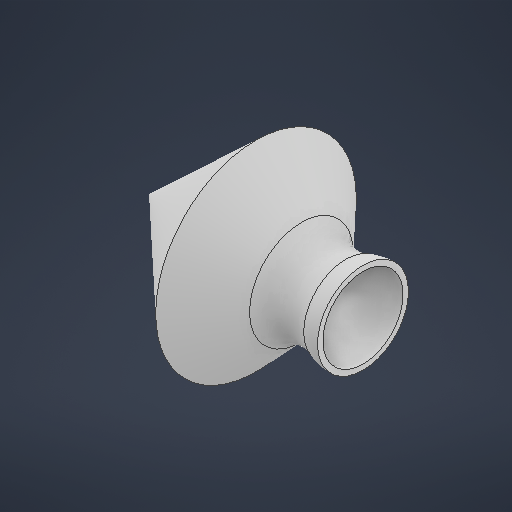
# Autodesk Inventor part: cabeza
Saved by Autodesk Inventor 2026.2 (Build 302298000, 298)
## iProperties
Created: 2026-05-21
Part Number: cabeza
Material: Generic
Document SubType Name: Modeling
Designer: juand
Density: 1 g/cm^3
Appearance: Default
Author: juand
Autodesk Inventor part; units mm, degrees
ref_plane "YZ Plane" through (0, 0, 0) normal (1, 0, 0) x (0, 1, 0)
ref_plane "XZ Plane" through (0, 0, 0) normal (0, 1, 0) x (-1, 0, 0)
ref_plane "XY Plane" through (0, 0, 0) normal (0, 0, 1) x (1, 0, 0)
sketch "Sketch1" plane through (0, 0, 0) normal (0, 0, 1) x (1, 0, 0)
  line L0 (0, 0) -> (0, 15) construction
  line L1 (0, 0) -> (-80, 0)
  arc A0 (0, 15) -> (-15, 0) centre (0, 0) ccw
  line L2 (-12.5483, 8.2182) -> (-40, 37.5)
  line L3 (-40, 37.5) -> (-80, 0)
  line L4 (-40, 0) -> (-40, 37.5) construction
  line L5 (-13.0868, 7.3305) -> (-40.0456, 36.0865)
  line L6 (-40.0456, 36.0865) -> (-78.5379, 0)
  arc A1 (0, 17) -> (-17, 0) centre (0, 0) ccw
  line L7 (0, 15) -> (0, 17)
  point P0 (-13.951, 9.7144)
  point P1 (-14.5134, 8.8522)
  dimension "d0" = 15
  dimension "d1" = 75
  dimension "d2" = 80
  dimension "d3" = 90
  dimension "d4" = 1
  dimension "d5" = 2
  constraints: 16 end point, 6 point on circle, 3 point on line, 3 vertical, 2 centre point, 2 coincident, 1 horizontal, 1 midpoint, 1 other
  measures "d0" radius of A0
  measures "d1" diameter of L2.end L1
  measures "d2" distance of L0.start L1.end
  measures "d3" angle of L3 L2
  measures "d4" distance between parallel lines of L2 L5
  measures "d5" radial gap between concentric circles of A0 A1
revolve "Revolution1" add sketch "Sketch1" angle 360 about axis through (0, 0, 0) along (-1, 0, 0) contours L1 A1 L5 A0 | L5 A1 L2 A0 | L1 L3 L2 A1 L5 L6 | L2 A1 L7 A0
fillet "Fillet1" radius 15 1 edges at (-13.951, -9.7144, 0)
body "Solid1"
